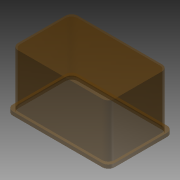
# Autodesk Inventor part: cuva
Saved by Autodesk Inventor 2015 SP1 (Build 190203100, 203)
## iProperties
Created: 2015-04-23
Part Number: cuva
Material: Polycarbonate, Smoke
Document SubType Name: Modeling
Designer: ubik
Density: 1.2 g/cm^3
Appearance: Polycarbonate - Smoked
Author: ubik
Autodesk Inventor part; units mm, degrees
ref_plane "YZ Plane" through (0, 0, 0) normal (1, 0, 0) x (0, 1, 0)
ref_plane "XZ Plane" through (0, 0, 0) normal (0, 1, 0) x (-1, 0, 0)
ref_plane "XY Plane" through (0, 0, 0) normal (0, 0, 1) x (1, 0, 0)
sketch "Sketch1" plane through (0, 0, 0) normal (0, 0, 1) x (1, 0, 0)
  line L0 (0, 0) -> (187.5, 0)
  line L1 (187.5, 0) -> (187.5, 116)
  line L2 (187.5, 116) -> (0, 116)
  line L3 (0, 116) -> (0, 0)
  line L4 (-5, -5) -> (192.5, -5)
  line L5 (192.5, -5) -> (192.5, 121)
  line L6 (192.5, 121) -> (-5, 121)
  line L7 (-5, 121) -> (-5, -5)
  dimension "d0" = 116
  dimension "d1" = 187.5
  dimension "d2" = 5
  dimension "d3" = 5
  dimension "d4" = 5
  dimension "d5" = 5
  constraints: 16 end point, 4 parallel, 2 horizontal, 2 perpendicular
  measures "d0" distance of L2.end L0.start
  measures "d1" distance of L0.start L0.end
  measures "d2" distance between parallel lines of L3 L7
  measures "d3" distance between parallel lines of L0 L4
  measures "d4" distance between parallel lines of L1 L5
  measures "d5" distance between parallel lines of L2 L6
extrude "Extrusion1" add sketch "Sketch1" along normal blind 7
fillet "Fillet1" radius 12 8 edges at (-5, -5, 3.5) (-5, 121, 3.5) (192.5, 121, 3.5) (192.5, -5, 3.5) (0, 0, 3.5) (187.5, 116, 3.5) (0, 116, 3.5) (187.5, 0, 3.5)
sketch "Sketch2" plane through (0, 0, 7) normal (0, 0, 1) x (1, 0, 0)
  line L0 (0, 12) -> (0, 104) projected
  arc A0 (12, 116) -> (0, 104) centre (12, 104) ccw projected
  arc A1 (0, 12) -> (12, 0) centre (12, 12) ccw projected
  line L1 (175.5, 0) -> (12, 0) projected
  line L2 (12, 116) -> (175.5, 116) projected
  arc A2 (187.5, 104) -> (175.5, 116) centre (175.5, 104) ccw projected
  line L3 (187.5, 104) -> (187.5, 12) projected
  arc A3 (175.5, 0) -> (187.5, 12) centre (175.5, 12) ccw projected
  line L4 (14, 2) -> (173.5, 2)
  line L5 (185.5, 14) -> (185.5, 102)
  line L6 (173.5, 114) -> (14, 114)
  line L7 (2, 102) -> (2, 14)
  arc A4 (2, 14) -> (14, 2) centre (14, 14) ccw
  arc A5 (14, 114) -> (2, 102) centre (14, 102) ccw
  arc A6 (185.5, 102) -> (173.5, 114) centre (173.5, 102) ccw
  arc A7 (173.5, 2) -> (185.5, 14) centre (173.5, 14) ccw
  point P0 (0, 0)
  dimension "d9" = 2
  dimension "d10" = 2
  dimension "d11" = 2
  dimension "d12" = 2
  dimension "d13" = 12
  constraints: 8 end point, 8 point on circle, 8 tangent, 4 centre point, 3 equal radius, 2 parallel, 1 horizontal, 1 perpendicular
  measures "d9" distance between parallel lines of L3 L5
  measures "d10" distance between parallel lines of L1 L4
  measures "d11" distance between parallel lines of L2 L6
  measures "d12" distance between parallel lines of L0 L7
  measures "d13" radius of A4
extrude "Extrusion2" add sketch "Sketch2" along normal blind 103
sketch "Sketch3" plane through (0, 0, 110) normal (0, 0, 1) x (1, 0, 0)
  arc A0 (2, 14) -> (14, 2) centre (14, 14) ccw projected
  line L0 (2, 14) -> (2, 102) projected
  line L1 (173.5, 2) -> (14, 2) projected
  arc A1 (14, 114) -> (2, 102) centre (14, 102) ccw projected
  line L2 (14, 114) -> (173.5, 114) projected
  arc A2 (185.5, 102) -> (173.5, 114) centre (173.5, 102) ccw projected
  line L3 (185.5, 102) -> (185.5, 14) projected
  arc A3 (173.5, 2) -> (185.5, 14) centre (173.5, 14) ccw projected
  point P0 (0, 0)
extrude "Extrusion3" add sketch "Sketch3" against normal blind 2
body "Solid1"
